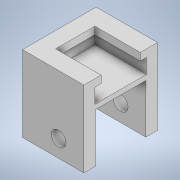
# Autodesk Inventor part: baseA
Saved by Autodesk Inventor 2021.4 (Build 254397000, 397)
## iProperties
Created: 2023-11-06
Part Number: baseA
Material: 一般
Document SubType Name: Modeling
Designer: ryusei
Density: 1 g/cm^3
Appearance: 既定
Author: ryusei
Autodesk Inventor part; units mm, degrees
ref_plane "YZ Plane" through (0, 0, 0) normal (1, 0, 0) x (0, 1, 0)
ref_plane "XZ Plane" through (0, 0, 0) normal (0, 1, 0) x (-1, 0, 0)
ref_plane "XY Plane" through (0, 0, 0) normal (0, 0, 1) x (1, 0, 0)
sketch "スケッチ1" plane through (0, 0, 0) normal (0, 1, 0) x (-1, 0, 0)
  line L0 (-12.5, -15) -> (12.5, -15)
  line L1 (12.5, -15) -> (12.5, 15)
  line L2 (12.5, 15) -> (-12.5, 15)
  line L3 (-12.5, 15) -> (-12.5, -15)
  line L4 (-12.5, -15) -> (12.5, 15) construction
  line L5 (12.5, -15) -> (-12.5, 15) construction
  point P0 (0, 0)
  dimension "d0" = 25
  dimension "d1" = 30
  constraints: 12 end point, 2 midpoint, 2 parallel, 1 horizontal, 1 perpendicular
  measures "d0" distance of L2.end L1.end
  measures "d1" distance of L1.end L0.end
extrude "押し出し1" add sketch "スケッチ1" along normal blind 25
sketch "スケッチ2" plane through (0, 0, 0) normal (0, -1, 0) x (1, 0, 0)
  line L0 (12.5, 15) -> (12.5, -15) projected
  line L1 (12.5, -10.25) -> (-8, -10.25)
  line L2 (-8, -10.25) -> (-8, 10.25)
  line L3 (-8, 10.25) -> (12.5, 10.25)
  line L4 (12.5, 10.25) -> (12.5, -10.25)
  line L5 (12.5, -15) -> (-12.5, -15) projected
  point P0 (0, 0)
  point P1 (12.5, 10.25)
  dimension "d4" = 20.5
  dimension "d5" = 20.5
  dimension "d22" = 10.25
  constraints: 8 end point, 2 parallel, 1 horizontal, 1 perpendicular, 1 point on line
  measures "d4" distance of L2.end L3.end
  measures "d5" distance of L1.end L2.end
  measures "d22" distance from line of L1 point (0, 0)
extrude "押し出し2" cut sketch "スケッチ2" against normal blind 20
sketch "スケッチ4" plane through (12.5, 0, -15) normal (0, 0, -1) x (-1, 0, 0)
  line L0 (0, 0) -> (25, 0) projected
  line L1 (0, 0) -> (0, 25) projected
  point P0 (12.5, 0)
  point P1 (10.25, 7)
  dimension "d12" = 7
  dimension "d13" = 10.25
  measures "d12" distance from line of L0 point (10.25, 7)
  measures "d13" distance from line of L1 point (10.25, 7)
hole "穴1" at (2.25, 7, -15) direction (0, 0, 1) diameter 6 end through all
sketch "スケッチ6" plane through (0, 25, 0) normal (0, 1, 0) x (1, 0, 0)
  line L0 (-12.5, 15) -> (-12.5, -15) projected
  line L1 (12.5, -15) -> (12.5, -10.25) projected
  line L2 (-12.5, 15) -> (12.5, 15)
  line L3 (12.5, 15) -> (12.5, -15)
  line L4 (12.5, -15) -> (-12.5, -15)
  line L5 (-12.5, -15) -> (-12.5, 15)
  point P0 (0, 0)
  constraints: 8 end point, 2 parallel, 1 horizontal, 1 perpendicular
extrude "押し出し5" add sketch "スケッチ6" along normal blind 6
sketch "スケッチ8" plane through (12.5, 0, -10.25) normal (1, 0, 0) x (0, 0, -1)
  line L0 (-20.75, 28) -> (0.25, 28)
  line L1 (0.25, 28) -> (0.25, 22)
  line L2 (0.25, 22) -> (-20.75, 22)
  line L3 (-20.75, 22) -> (-20.75, 28)
  line L4 (-20.5, 20) -> (0, 20) projected
  point P0 (-10.25, 0)
  dimension "d37" = 21
  dimension "d38" = 6
  dimension "d39" = 10.5
  dimension "d40" = 2
  constraints: 8 end point, 2 parallel, 1 horizontal, 1 perpendicular
  measures "d37" distance of L1.end L2.end
  measures "d38" distance of L2.end L0.start
  measures "d39" distance from line of point (-10.25, 0) L3
  measures "d40" distance between parallel lines of L4 L2
extrude "押し出し7" cut sketch "スケッチ8" against normal blind 21
sketch "スケッチ9" plane through (12.5, 0, -10.25) normal (1, 0, 0) x (0, 0, -1)
  line L0 (-18.25, 31) -> (-2.25, 31)
  line L1 (-2.25, 31) -> (-2.25, 28)
  line L2 (-2.25, 28) -> (-18.25, 28)
  line L3 (-18.25, 28) -> (-18.25, 31)
  line L4 (-25.25, 31) -> (4.75, 31) projected
  point P0 (-10.25, 0)
  dimension "d43" = 16
  dimension "d44" = 3
  dimension "d45" = 0
  dimension "d46" = 8
  constraints: 8 end point, 2 parallel, 1 horizontal, 1 perpendicular
  measures "d43" distance of L1.end L2.end
  measures "d44" distance of L0.end L1.end
  measures "d45" distance between parallel lines of L4 L0
  measures "d46" distance from line of point (-10.25, 0) L1
extrude "押し出し8" cut sketch "スケッチ9" against normal blind 18.5
